Autodesk Inventor part; units mm, degrees
(part 2 of 2)
sketch "スケッチ9" plane through (0, 6.3499, -121.1637) normal (-1, 0, 0) x (0, -0.052336, 0.9986295)
  circle A0 centre (121.33, 0) radius 8 projected
  line L0 (-0.2546, 4.5097) -> (1.6876, 3.599) projected
  arc A1 (1.6876, -3.599) -> (1.6876, 3.599) centre (0, 0) ccw projected
  line L1 (1.6876, -3.599) -> (-0.2546, -4.5097) projected
  arc A2 (-0.2546, -4.5097) -> (-0.0599, -8.2241) centre (121.33, 0) ccw projected
  line L2 (-0.0599, -8.2241) -> (1.9668, -8.9268) projected
  arc A3 (2.7192, -16.0853) -> (1.9668, -8.9268) centre (0.6647, -12.6824) ccw projected
  line L3 (2.7192, -16.0853) -> (0.8829, -17.194) projected
  arc A4 (0.8829, -17.194) -> (1.4648, -20.8677) centre (121.33, 0) ccw projected
  line L4 (1.4648, -20.8677) -> (3.5538, -21.3547) projected
  arc A5 (5.0503, -28.3954) -> (3.5538, -21.3547) centre (2.6514, -25.2259) ccw projected
  line L5 (5.0503, -28.3954) -> (3.34, -29.69) projected
  arc A6 (3.34, -29.69) -> (4.3027, -33.2828) centre (121.33, 0) ccw projected
  line L6 (4.3027, -33.2828) -> (6.4311, -33.5487) projected
  arc A7 (8.6554, -40.3944) -> (6.4311, -33.5487) centre (5.9383, -37.493) ccw projected
  line L7 (8.6554, -40.3944) -> (7.0898, -41.8606) projected
  arc A8 (7.0898, -41.8606) -> (8.4227, -45.3331) centre (121.33, 0) ccw projected
  line L8 (8.4227, -45.3331) -> (10.5674, -45.3751) projected
  arc A9 (13.495, -51.9508) -> (10.5674, -45.3751) centre (10.4895, -49.3494) ccw projected
  line L9 (13.495, -51.9508) -> (12.0912, -53.5727) projected
  arc A10 (12.0912, -53.5727) -> (13.7799, -56.8868) centre (121.33, 0) ccw projected
  line L10 (13.7799, -56.8868) -> (15.9171, -56.7044) projected
  arc A11 (19.5161, -62.938) -> (15.9171, -56.7044) centre (16.2551, -60.665) ccw projected
  line L11 (19.5161, -62.938) -> (18.2895, -64.6977) projected
  arc A12 (18.2895, -64.6977) -> (20.3153, -67.8172) centre (121.33, 0) ccw projected
  line L12 (20.3153, -67.8172) -> (22.4218, -67.4124) projected
  arc A13 (26.6527, -73.2357) -> (22.4218, -67.4124) centre (23.172, -71.316) ccw projected
  line L13 (26.6527, -73.2357) -> (25.6167, -75.114) projected
  arc A14 (25.6167, -75.114) -> (27.9575, -78.0046) centre (121.33, 0) ccw projected
  line L14 (27.9575, -78.0046) -> (30.0101, -77.3818) projected
  arc A15 (34.8265, -82.731) -> (30.0101, -77.3818) centre (31.1642, -81.1856) ccw projected
  line L15 (34.8265, -82.731) -> (33.9926, -84.7073) projected
  arc A16 (33.9926, -84.7073) -> (36.6227, -87.3374) centre (121.33, 0) ccw projected
  line L16 (36.6227, -87.3374) -> (38.599, -86.5035) projected
  arc A17 (43.9482, -91.3199) -> (38.599, -86.5035) centre (40.1444, -90.1658) ccw projected
  line L17 (43.9482, -91.3199) -> (43.3254, -93.3725) projected
  arc A18 (43.3254, -93.3725) -> (46.216, -95.7133) centre (121.33, 0) ccw projected
  line L18 (46.216, -95.7133) -> (48.0943, -94.6773) projected
  arc A19 (53.9176, -98.9082) -> (48.0943, -94.6773) centre (50.014, -98.158) ccw projected
  line L19 (53.9176, -98.9082) -> (53.5128, -101.0147) projected
  arc A20 (53.5128, -101.0147) -> (56.6323, -103.0405) centre (121.33, 0) ccw projected
  line L20 (56.6323, -103.0405) -> (58.392, -101.8139) projected
  arc A21 (64.6256, -105.4129) -> (58.392, -101.8139) centre (60.665, -105.0749) ccw projected
  line L21 (64.6256, -105.4129) -> (64.4432, -107.5501) projected
  arc A22 (64.4432, -107.5501) -> (67.7573, -109.2388) centre (121.33, 0) ccw projected
  line L22 (67.7573, -109.2388) -> (69.3792, -107.835) projected
  arc A23 (75.9549, -110.7626) -> (69.3792, -107.835) centre (71.9806, -110.8405) ccw projected
  line L23 (75.9549, -110.7626) -> (75.9969, -112.9073) projected
  arc A24 (75.9969, -112.9073) -> (79.4694, -114.2402) centre (121.33, 0) ccw projected
  line L24 (79.4694, -114.2402) -> (80.9356, -112.6746) projected
  arc A25 (87.7813, -114.8989) -> (80.9356, -112.6746) centre (83.837, -115.3917) ccw projected
  line L25 (87.7813, -114.8989) -> (88.0472, -117.0273) projected
  arc A26 (88.0472, -117.0273) -> (91.64, -117.99) centre (121.33, 0) ccw projected
  line L26 (91.64, -117.99) -> (92.9346, -116.2797) projected
  arc A27 (99.9753, -117.7762) -> (92.9346, -116.2797) centre (96.1041, -118.6786) ccw projected
  line L27 (99.9753, -117.7762) -> (100.4623, -119.8652) projected
  arc A28 (100.4623, -119.8652) -> (104.136, -120.4471) centre (121.33, 0) ccw projected
  line L28 (104.136, -120.4471) -> (105.2447, -118.6108) projected
  arc A29 (112.4032, -119.3632) -> (105.2447, -118.6108) centre (108.6476, -120.6653) ccw projected
  line L29 (112.4032, -119.3632) -> (113.1059, -121.3899) projected
  arc A30 (113.1059, -121.3899) -> (116.8203, -121.5846) centre (121.33, 0) ccw projected
  line L30 (116.8203, -121.5846) -> (117.731, -119.6424) projected
  arc A31 (124.929, -119.6424) -> (117.731, -119.6424) centre (121.33, -121.33) ccw projected
  line L31 (124.929, -119.6424) -> (125.8397, -121.5846) projected
  arc A32 (125.8397, -121.5846) -> (129.5541, -121.3899) centre (121.33, 0) ccw projected
  line L32 (129.5541, -121.3899) -> (130.2568, -119.3632) projected
  arc A33 (137.4153, -118.6108) -> (130.2568, -119.3632) centre (134.0124, -120.6653) ccw projected
  line L33 (137.4153, -118.6108) -> (138.524, -120.4471) projected
  arc A34 (138.524, -120.4471) -> (142.1977, -119.8652) centre (121.33, 0) ccw projected
  line L34 (142.1977, -119.8652) -> (142.6847, -117.7762) projected
  arc A35 (149.7254, -116.2797) -> (142.6847, -117.7762) centre (146.5559, -118.6786) ccw projected
  line L35 (149.7254, -116.2797) -> (151.02, -117.99) projected
  arc A36 (151.02, -117.99) -> (154.6128, -117.0273) centre (121.33, 0) ccw projected
  line L36 (154.6128, -117.0273) -> (154.8787, -114.8989) projected
  arc A37 (161.7244, -112.6746) -> (154.8787, -114.8989) centre (158.823, -115.3917) ccw projected
  line L37 (161.7244, -112.6746) -> (163.1906, -114.2402) projected
  arc A38 (163.1906, -114.2402) -> (166.6631, -112.9073) centre (121.33, 0) ccw projected
  line L38 (166.6631, -112.9073) -> (166.7051, -110.7626) projected
  arc A39 (173.2808, -107.835) -> (166.7051, -110.7626) centre (170.6794, -110.8405) ccw projected
  line L39 (173.2808, -107.835) -> (174.9027, -109.2388) projected
  arc A40 (174.9027, -109.2388) -> (178.2168, -107.5501) centre (121.33, 0) ccw projected
  line L40 (178.2168, -107.5501) -> (178.0344, -105.4129) projected
  arc A41 (184.268, -101.8139) -> (178.0344, -105.4129) centre (181.995, -105.0749) ccw projected
  line L41 (184.268, -101.8139) -> (186.0277, -103.0405) projected
  arc A42 (186.0277, -103.0405) -> (189.1472, -101.0147) centre (121.33, 0) ccw projected
  line L42 (189.1472, -101.0147) -> (188.7424, -98.9082) projected
  arc A43 (194.5657, -94.6773) -> (188.7424, -98.9082) centre (192.646, -98.158) ccw projected
  line L43 (194.5657, -94.6773) -> (196.444, -95.7133) projected
  arc A44 (196.444, -95.7133) -> (199.3346, -93.3725) centre (121.33, 0) ccw projected
  line L44 (199.3346, -93.3725) -> (198.7118, -91.3199) projected
  arc A45 (204.061, -86.5035) -> (198.7118, -91.3199) centre (202.5156, -90.1658) ccw projected
  line L45 (204.061, -86.5035) -> (206.0373, -87.3374) projected
  arc A46 (206.0373, -87.3374) -> (208.6674, -84.7073) centre (121.33, 0) ccw projected
  line L46 (208.6674, -84.7073) -> (207.8335, -82.731) projected
  arc A47 (212.6499, -77.3818) -> (207.8335, -82.731) centre (211.4958, -81.1856) ccw projected
  line L47 (212.6499, -77.3818) -> (214.7025, -78.0046) projected
  arc A48 (214.7025, -78.0046) -> (217.0433, -75.114) centre (121.33, 0) ccw projected
  line L48 (217.0433, -75.114) -> (216.0073, -73.2357) projected
  arc A49 (220.2382, -67.4124) -> (216.0073, -73.2357) centre (219.488, -71.316) ccw projected
  line L49 (220.2382, -67.4124) -> (222.3447, -67.8172) projected
  arc A50 (222.3447, -67.8172) -> (224.3705, -64.6977) centre (121.33, 0) ccw projected
  line L50 (224.3705, -64.6977) -> (223.1439, -62.938) projected
  arc A51 (226.7429, -56.7044) -> (223.1439, -62.938) centre (226.4049, -60.665) ccw projected
  line L51 (226.7429, -56.7044) -> (228.8801, -56.8868) projected
  arc A52 (228.8801, -56.8868) -> (230.5688, -53.5727) centre (121.33, 0) ccw projected
  line L52 (230.5688, -53.5727) -> (229.165, -51.9508) projected
  arc A53 (232.0926, -45.3751) -> (229.165, -51.9508) centre (232.1705, -49.3494) ccw projected
  line L53 (232.0926, -45.3751) -> (234.2373, -45.3331) projected
  arc A54 (234.2373, -45.3331) -> (235.5702, -41.8606) centre (121.33, 0) ccw projected
  line L54 (235.5702, -41.8606) -> (234.0046, -40.3944) projected
  arc A55 (236.2289, -33.5487) -> (234.0046, -40.3944) centre (236.7217, -37.493) ccw projected
  line L55 (236.2289, -33.5487) -> (238.3573, -33.2828) projected
  arc A56 (238.3573, -33.2828) -> (239.32, -29.69) centre (121.33, 0) ccw projected
  line L56 (239.32, -29.69) -> (237.6097, -28.3954) projected
  arc A57 (239.1062, -21.3547) -> (237.6097, -28.3954) centre (240.0086, -25.2259) ccw projected
  line L57 (239.1062, -21.3547) -> (241.1952, -20.8677) projected
  arc A58 (241.1952, -20.8677) -> (241.7771, -17.194) centre (121.33, 0) ccw projected
  line L58 (241.7771, -17.194) -> (239.9408, -16.0853) projected
  arc A59 (240.6932, -8.9268) -> (239.9408, -16.0853) centre (241.9953, -12.6824) ccw projected
  line L59 (240.6932, -8.9268) -> (242.7199, -8.2241) projected
  arc A60 (242.7199, -8.2241) -> (242.9146, -4.5097) centre (121.33, 0) ccw projected
  line L60 (242.9146, -4.5097) -> (240.9724, -3.599) projected
  arc A61 (240.9724, 3.599) -> (240.9724, -3.599) centre (242.66, 0) ccw projected
  line L61 (240.9724, 3.599) -> (242.9146, 4.5097) projected
  arc A62 (242.9146, 4.5097) -> (242.7199, 8.2241) centre (121.33, 0) ccw projected
  line L62 (242.7199, 8.2241) -> (240.6932, 8.9268) projected
  arc A63 (239.9408, 16.0853) -> (240.6932, 8.9268) centre (241.9953, 12.6824) ccw projected
  line L63 (239.9408, 16.0853) -> (241.7771, 17.194) projected
  arc A64 (241.7771, 17.194) -> (241.1952, 20.8677) centre (121.33, 0) ccw projected
  line L64 (241.1952, 20.8677) -> (239.1062, 21.3547) projected
  arc A65 (237.6097, 28.3954) -> (239.1062, 21.3547) centre (240.0086, 25.2259) ccw projected
  line L65 (237.6097, 28.3954) -> (239.32, 29.69) projected
  arc A66 (239.32, 29.69) -> (238.3573, 33.2828) centre (121.33, 0) ccw projected
  line L66 (238.3573, 33.2828) -> (236.2289, 33.5487) projected
  arc A67 (234.0046, 40.3944) -> (236.2289, 33.5487) centre (236.7217, 37.493) ccw projected
  line L67 (234.0046, 40.3944) -> (235.5702, 41.8606) projected
  arc A68 (235.5702, 41.8606) -> (234.2373, 45.3331) centre (121.33, 0) ccw projected
  line L68 (234.2373, 45.3331) -> (232.0926, 45.3751) projected
  arc A69 (229.165, 51.9508) -> (232.0926, 45.3751) centre (232.1705, 49.3494) ccw projected
  line L69 (229.165, 51.9508) -> (230.5688, 53.5727) projected
  arc A70 (230.5688, 53.5727) -> (228.8801, 56.8868) centre (121.33, 0) ccw projected
  line L70 (228.8801, 56.8868) -> (226.7429, 56.7044) projected
  arc A71 (223.1439, 62.938) -> (226.7429, 56.7044) centre (226.4049, 60.665) ccw projected
  line L71 (223.1439, 62.938) -> (224.3705, 64.6977) projected
  arc A72 (224.3705, 64.6977) -> (222.3447, 67.8172) centre (121.33, 0) ccw projected
  line L72 (222.3447, 67.8172) -> (220.2382, 67.4124) projected
  arc A73 (216.0073, 73.2357) -> (220.2382, 67.4124) centre (219.488, 71.316) ccw projected
  line L73 (216.0073, 73.2357) -> (217.0433, 75.114) projected
  arc A74 (217.0433, 75.114) -> (214.7025, 78.0046) centre (121.33, 0) ccw projected
  line L74 (214.7025, 78.0046) -> (212.6499, 77.3818) projected
  arc A75 (207.8335, 82.731) -> (212.6499, 77.3818) centre (211.4958, 81.1856) ccw projected
  line L75 (207.8335, 82.731) -> (208.6674, 84.7073) projected
  arc A76 (208.6674, 84.7073) -> (206.0373, 87.3374) centre (121.33, 0) ccw projected
  line L76 (206.0373, 87.3374) -> (204.061, 86.5035) projected
  arc A77 (198.7118, 91.3199) -> (204.061, 86.5035) centre (202.5156, 90.1658) ccw projected
  line L77 (198.7118, 91.3199) -> (199.3346, 93.3725) projected
  arc A78 (199.3346, 93.3725) -> (196.444, 95.7133) centre (121.33, 0) ccw projected
  line L78 (196.444, 95.7133) -> (194.5657, 94.6773) projected
  arc A79 (188.7424, 98.9082) -> (194.5657, 94.6773) centre (192.646, 98.158) ccw projected
  line L79 (188.7424, 98.9082) -> (189.1472, 101.0147) projected
  arc A80 (189.1472, 101.0147) -> (186.0277, 103.0405) centre (121.33, 0) ccw projected
  line L80 (186.0277, 103.0405) -> (184.268, 101.8139) projected
  arc A81 (178.0344, 105.4129) -> (184.268, 101.8139) centre (181.995, 105.0749) ccw projected
  line L81 (178.0344, 105.4129) -> (178.2168, 107.5501) projected
  arc A82 (178.2168, 107.5501) -> (174.9027, 109.2388) centre (121.33, 0) ccw projected
  line L82 (174.9027, 109.2388) -> (173.2808, 107.835) projected
  arc A83 (166.7051, 110.7626) -> (173.2808, 107.835) centre (170.6794, 110.8405) ccw projected
  line L83 (166.7051, 110.7626) -> (166.6631, 112.9073) projected
  arc A84 (166.6631, 112.9073) -> (163.1906, 114.2402) centre (121.33, 0) ccw projected
  line L84 (163.1906, 114.2402) -> (161.7244, 112.6746) projected
  arc A85 (154.8787, 114.8989) -> (161.7244, 112.6746) centre (158.823, 115.3917) ccw projected
  line L85 (154.8787, 114.8989) -> (154.6128, 117.0273) projected
  arc A86 (154.6128, 117.0273) -> (151.02, 117.99) centre (121.33, 0) ccw projected
  line L86 (151.02, 117.99) -> (149.7254, 116.2797) projected
  arc A87 (142.6847, 117.7762) -> (149.7254, 116.2797) centre (146.5559, 118.6786) ccw projected
  line L87 (142.6847, 117.7762) -> (142.1977, 119.8652) projected
  arc A88 (142.1977, 119.8652) -> (138.524, 120.4471) centre (121.33, 0) ccw projected
  line L88 (138.524, 120.4471) -> (137.4153, 118.6108) projected
  arc A89 (130.2568, 119.3632) -> (137.4153, 118.6108) centre (134.0124, 120.6653) ccw projected
  line L89 (130.2568, 119.3632) -> (129.5541, 121.3899) projected
  arc A90 (129.5541, 121.3899) -> (125.8397, 121.5846) centre (121.33, 0) ccw projected
  line L90 (125.8397, 121.5846) -> (124.929, 119.6424) projected
  arc A91 (117.731, 119.6424) -> (124.929, 119.6424) centre (121.33, 121.33) ccw projected
  line L91 (117.731, 119.6424) -> (116.8203, 121.5846) projected
  arc A92 (116.8203, 121.5846) -> (113.1059, 121.3899) centre (121.33, 0) ccw projected
  line L92 (113.1059, 121.3899) -> (112.4032, 119.3632) projected
  arc A93 (105.2447, 118.6108) -> (112.4032, 119.3632) centre (108.6476, 120.6653) ccw projected
  line L93 (105.2447, 118.6108) -> (104.136, 120.4471) projected
  arc A94 (104.136, 120.4471) -> (100.4623, 119.8652) centre (121.33, 0) ccw projected
  line L94 (100.4623, 119.8652) -> (99.9753, 117.7762) projected
  arc A95 (92.9346, 116.2797) -> (99.9753, 117.7762) centre (96.1041, 118.6786) ccw projected
  line L95 (92.9346, 116.2797) -> (91.64, 117.99) projected
  arc A96 (91.64, 117.99) -> (88.0472, 117.0273) centre (121.33, 0) ccw projected
  line L96 (88.0472, 117.0273) -> (87.7813, 114.8989) projected
  arc A97 (80.9356, 112.6746) -> (87.7813, 114.8989) centre (83.837, 115.3917) ccw projected
  line L97 (80.9356, 112.6746) -> (79.4694, 114.2402) projected
  arc A98 (79.4694, 114.2402) -> (75.9969, 112.9073) centre (121.33, 0) ccw projected
  line L98 (75.9969, 112.9073) -> (75.9549, 110.7626) projected
  arc A99 (69.3792, 107.835) -> (75.9549, 110.7626) centre (71.9806, 110.8405) ccw projected
  line L99 (69.3792, 107.835) -> (67.7573, 109.2388) projected
  arc A100 (67.7573, 109.2388) -> (64.4432, 107.5501) centre (121.33, 0) ccw projected
  line L100 (64.4432, 107.5501) -> (64.6256, 105.4129) projected
  arc A101 (58.392, 101.8139) -> (64.6256, 105.4129) centre (60.665, 105.0749) ccw projected
  line L101 (58.392, 101.8139) -> (56.6323, 103.0405) projected
  arc A102 (56.6323, 103.0405) -> (53.5128, 101.0147) centre (121.33, 0) ccw projected
  line L102 (53.5128, 101.0147) -> (53.9176, 98.9082) projected
  arc A103 (48.0943, 94.6773) -> (53.9176, 98.9082) centre (50.014, 98.158) ccw projected
  line L103 (48.0943, 94.6773) -> (46.216, 95.7133) projected
  arc A104 (46.216, 95.7133) -> (43.3254, 93.3725) centre (121.33, 0) ccw projected
  line L104 (43.3254, 93.3725) -> (43.9482, 91.3199) projected
  arc A105 (38.599, 86.5035) -> (43.9482, 91.3199) centre (40.1444, 90.1658) ccw projected
  line L105 (38.599, 86.5035) -> (36.6227, 87.3374) projected
  arc A106 (36.6227, 87.3374) -> (33.9926, 84.7073) centre (121.33, 0) ccw projected
  line L106 (33.9926, 84.7073) -> (34.8265, 82.731) projected
  arc A107 (30.0101, 77.3818) -> (34.8265, 82.731) centre (31.1642, 81.1856) ccw projected
  line L107 (30.0101, 77.3818) -> (27.9575, 78.0046) projected
  arc A108 (27.9575, 78.0046) -> (25.6167, 75.114) centre (121.33, 0) ccw projected
  line L108 (25.6167, 75.114) -> (26.6527, 73.2357) projected
  arc A109 (22.4218, 67.4124) -> (26.6527, 73.2357) centre (23.172, 71.316) ccw projected
  line L109 (22.4218, 67.4124) -> (20.3153, 67.8172) projected
  arc A110 (20.3153, 67.8172) -> (18.2895, 64.6977) centre (121.33, 0) ccw projected
  line L110 (18.2895, 64.6977) -> (19.5161, 62.938) projected
  arc A111 (15.9171, 56.7044) -> (19.5161, 62.938) centre (16.2551, 60.665) ccw projected
  line L111 (15.9171, 56.7044) -> (13.7799, 56.8868) projected
  arc A112 (13.7799, 56.8868) -> (12.0912, 53.5727) centre (121.33, 0) ccw projected
  line L112 (12.0912, 53.5727) -> (13.495, 51.9508) projected
  arc A113 (10.5674, 45.3751) -> (13.495, 51.9508) centre (10.4895, 49.3494) ccw projected
  line L113 (10.5674, 45.3751) -> (8.4227, 45.3331) projected
  arc A114 (8.4227, 45.3331) -> (7.0898, 41.8606) centre (121.33, 0) ccw projected
  line L114 (7.0898, 41.8606) -> (8.6554, 40.3944) projected
  arc A115 (6.4311, 33.5487) -> (8.6554, 40.3944) centre (5.9383, 37.493) ccw projected
  line L115 (6.4311, 33.5487) -> (4.3027, 33.2828) projected
  arc A116 (4.3027, 33.2828) -> (3.34, 29.69) centre (121.33, 0) ccw projected
  line L116 (3.34, 29.69) -> (5.0503, 28.3954) projected
  arc A117 (3.5538, 21.3547) -> (5.0503, 28.3954) centre (2.6514, 25.2259) ccw projected
  line L117 (3.5538, 21.3547) -> (1.4648, 20.8677) projected
  arc A118 (1.4648, 20.8677) -> (0.8829, 17.194) centre (121.33, 0) ccw projected
  line L118 (0.8829, 17.194) -> (2.7192, 16.0853) projected
  arc A119 (1.9668, 8.9268) -> (2.7192, 16.0853) centre (0.6647, 12.6824) ccw projected
  line L119 (1.9668, 8.9268) -> (-0.0599, 8.2241) projected
  arc A120 (-0.0599, 8.2241) -> (-0.2546, 4.5097) centre (121.33, 0) ccw projected
pattern_circular "円形状パターン1" count 6 over 360 about axis through (7.2, 0, 0) along (-1, 0, 0) of "押し出し8"
sketch "スケッチ10" plane through (5, 0, 0) normal (1, 0, 0) x (0, 0, -1)
  circle A0 centre (-12.6339, 79.7672) radius 11
  circle A1 centre (-43.7637, 54.0436) radius 17.5 projected
  circle A2 centre (24.9213, 64.9223) radius 17.5 projected
  line L0 (-43.7637, 54.0436) -> (24.9213, 64.9223)
  point P0 (0, 0)
  dimension "d32" = 22
  constraints: 2 end point, 1 centre point
  measures "d32" diameter of A0
extrude "押し出し9" cut sketch "スケッチ10" against normal through all contours A0
pattern_circular "円形状パターン2" count 6 over 360 about axis through (7.2, 0, 0) along (-1, 0, 0) of "押し出し9"
fillet "フィレット1" radius 2 1 edges at (5, -16.4037, 103.5686)
fillet "フィレット2" radius 2 2 edges at (7.2, -6.2574, 39.5075) (5, -6.2574, 39.5075)
sketch "スケッチ11" plane through (7.2, 0, 0) normal (1, 0, 0) x (0, 0, -1)
  circle A0 centre (-28.6287, 10.9895) radius 3.7496
  circle A1 centre (-75.3974, 28.9423) radius 11 projected
  line L0 (-75.3974, 28.9423) -> (0, 0)
  constraints: 2 end point, 1 centre point, 1 point on line
extrude "押し出し10" cut sketch "スケッチ11" against normal blind 9.4 contours A0 L0 | L0 A0
pattern_circular "円形状パターン3" count 12 over 360 about axis through (7.2, 0, 0) along (-1, 0, 0) of "押し出し10"
fillet "フィレット3" radius 2 6 edges at (5, 40.4436, 32.7506) (5, 48.5846, -18.6499) (5, -8.141, 51.4005) (5, -48.5846, 18.6499) (5, 8.141, -51.4005) (5, -40.4436, -32.7506)
body "Solid1"
